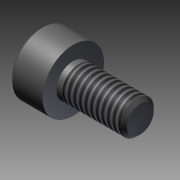
# Autodesk Inventor part: SCB3-6_1
Saved by Autodesk Inventor 2011 SP1 (Build 150282100, 282)
## iProperties
Created: 2015-02-01
Part Number: SCB3-6_1
Catalog Web Link: www.cadenas.de
Description: SCB_1-Hexagon Socket Head Cap Screws - Stainless Steel
Vendor: MISUMI
Document SubType Name: Modeling
Designer: PARTuser1
Manufacturer: MISUMI
Mass: 0.103858 g
Surface Area: 1.64097 cm^2
Volume: 0.103858 cm^3
Density: 1 g/cm^3
Category: PARTsolutions
Company: MISUMI
Title: SCB3-6_1
Author: Cadenas PARTsolutions
Comments: Hexagon Socket Head Cap Screws - Stainless Steel
PSOL_IDENT_0: {\\10.0.0.236\data_v8\23d-libs\misumi\metric\27_screws_nuts\scb.prj},158 {VTYP=3D},{NB=SCB3-6_1},{LI
PSOL_IDENT_1: NA=SCB3-6_1},{NN=SCB_1},{DATE=17.11.2014 07:44:00},{GEOMDATE=13.05.2010 00:00:00},{VERSION=},{LINEID=
PSOL_IDENT_2: 60},{LINESUBID=-1},{WBVAR=L}  {NB=SCB3-6_1},{LINA=SCB3-6_1},{KT=DUMMY},{PN=SCB3-6},{MAT=SUSXM7(30430
PSOL_IDENT_3: Stainless Steel)},{SC=A2-70},{M=3},{L=6},{LL=Full Thread},{L1=18},{TYPE=SCB},{M1=3.0},{M2=3.0},{L0=
PSOL_IDENT_4: 5,6,8,10,12,15,16,20,25,30},{MP=3x0.5},{P=0.5},{A=5.5},{E=3.0},{B=2.5},{V=0.30}
SUPPLIER: MISUMI
ARTICLENO: SCB3-6_1
BOMINFO: SCB3-6_1
CREATOR: CADENAS GmbH
Autodesk Inventor part; units mm, degrees
sketch "Sketch_1" plane through (0, 0, 0) normal (0, 0, 1) x (1, 0, 0)
  line L0 (6, 0) -> (-3, 0)
  line L1 (-3, 0) -> (-3, 2.45)
  line L2 (-3, 2.45) -> (-2.7, 2.75)
  line L3 (-2.7, 2.75) -> (0, 2.75)
  line L4 (0, 2.75) -> (0, 1.5)
  line L5 (0, 1.5) -> (5.6935, 1.5)
  line L6 (5.6935, 1.5) -> (6, 1.1935)
  line L7 (6, 1.1935) -> (6, 0)
  line L8 (6, 0) -> (-3, 0)
  constraints: 18 end point
revolve "Revolution1" add sketch "Sketch_1" angle 360 about axis through (6, 0, 0) along (1, 0, 0)
thread "Thread1" size "M3x0.5" class "6g" standard "ISO Metric profile" length 5.5 offset 0.5
sketch "Sketch_4" plane through (0, 0, 0) normal (0, 0, 1) x (1, 0, 0)
  line L0 (-1.1651, 0) -> (-3, 0)
  line L1 (-3, 0) -> (-3, 1.25)
  line L2 (-3, 1.25) -> (-1.5, 1.25)
  line L3 (-1.5, 1.25) -> (-1.1651, 0)
  line L4 (-1.1651, 0) -> (-3, 0)
  constraints: 10 end point
revolve "Revolution2" cut sketch "Sketch_4" angle 360 about axis through (-1.1651, 0, 0) along (1, 0, 0)
sketch "Sketch_3" plane through (-3, 0, 0) normal (1, 0, 0) x (0, 0, -1)
  line L0 (-1.25, 0.7217) -> (-1.25, -0.7217)
  line L1 (-1.25, -0.7217) -> (0, -1.4434)
  line L2 (0, -1.4434) -> (1.25, -0.7217)
  line L3 (1.25, -0.7217) -> (1.25, 0.7217)
  line L4 (1.25, 0.7217) -> (0, 1.4434)
  line L5 (0, 1.4434) -> (-1.25, 0.7217)
  constraints: 12 end point
extrude "Extrusion1" cut sketch "Sketch_3" along normal blind 1.5
ref_plane "nut_XY" through (6, 0, 0) normal (1, 0, 0) x (0, 0, -1)
ref_plane "nut_YZ" through (6, 0, 0) normal (0, 0, -1) x (0, 1, 0)
ref_plane "nut_ZX" through (6, 0, 0) normal (0, 1, 0) x (1, 0, 0)
ref_plane "bolt_XY" through (0, 0, 0) normal (1, 0, 0) x (0, 0, -1)
ref_plane "bolt_YZ" through (0, 0, 0) normal (0, 0, -1) x (0, 1, 0)
ref_plane "bolt_ZX" through (0, 0, 0) normal (0, 1, 0) x (1, 0, 0)
body "Solid1"
